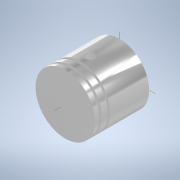
# Autodesk Inventor part: piston
Saved by Autodesk Inventor 2021.1 (Build 251245000, 245)
## iProperties
Created: 2020-08-31
Part Number: piston
Material: Aluminum 6061
Document SubType Name: Sheet Metal
Designer: Vamshi
Mass: 612.77 g
Surface Area: 445.688 cm^2
Volume: 226.952 cm^3
Density: 2.7 g/cm^3
Sheet Metal Rule: Default
Appearance: Aluminum - Flat
Author: Vamshi
Autodesk Inventor part; units mm, degrees
ref_plane "YZ Plane" through (0, 0, 0) normal (1, 0, 0) x (0, 1, 0)
ref_plane "XZ Plane" through (0, 0, 0) normal (0, 1, 0) x (-1, 0, 0)
ref_plane "XY Plane" through (0, 0, 0) normal (0, 0, 1) x (1, 0, 0)
sketch "Sketch1" plane through (0, 0, 0) normal (0, 0, 1) x (1, 0, 0)
  circle A0 centre (0, 0) radius 40.64
  dimension "d0" = 81.28
  constraints: 1 centre point, 1 coincident
  measures "d0" diameter of A0
extrude "Extrusion1" add sketch "Sketch1" along normal blind 81.28
sketch "Sketch2" plane through (0, 0, 0) normal (0, 1, 0) x (-1, 0, 0)
  line L0 (0, -16.256) -> (0, 97.536) construction
  line L1 (40.64, 81.28) -> (40.64, 0) construction
  line L2 (40.64, 0) -> (-40.64, 0) construction
  line L3 (-40.64, 0) -> (-40.64, 81.28) construction
  line L4 (-40.64, 81.28) -> (40.64, 81.28) construction
  line L5 (40.64, 81.28) -> (40.64, 0) construction
  line L6 (40.64, 0) -> (-40.64, 0) construction
  line L7 (-40.64, 0) -> (-40.64, 81.28) construction
  line L8 (-40.64, 81.28) -> (40.64, 81.28) construction
  line L9 (40.64, 81.28) -> (-40.64, 81.28) construction
  line L10 (40.64, 0) -> (-40.64, 0) construction
  line L11 (40.64, 0) -> (40.64, 81.28) projected
  line L12 (40.64, 68.58) -> (36.83, 68.58)
  line L13 (36.83, 68.58) -> (36.83, 64.77)
  line L14 (36.83, 64.77) -> (40.64, 64.77)
  line L15 (40.64, 64.77) -> (40.64, 68.58)
  line L16 (40.64, 57.15) -> (36.83, 57.15)
  line L17 (36.83, 57.15) -> (36.83, 53.34)
  line L18 (36.83, 53.34) -> (40.64, 53.34)
  line L19 (40.64, 53.34) -> (40.64, 57.15)
  line L20 (40.64, 0) -> (40.64, 81.28) projected
  line L21 (40.64, 81.28) -> (-40.64, 81.28) projected
  line L22 (0, 81.28) -> (40.64, 74.1141)
  line L23 (0, 0) -> (33.02, 0)
  line L24 (33.02, 0) -> (33.02, 25.4)
  line L25 (33.02, 25.4) -> (0, 25.4)
  line L26 (0, 25.4) -> (0, 0)
  line L27 (0, 25.4) -> (25.4, 25.4)
  line L28 (25.4, 25.4) -> (25.4, 60.96)
  line L29 (25.4, 60.96) -> (0, 60.96)
  line L30 (0, 60.96) -> (0, 25.4)
  dimension "d3" = 7.62
  dimension "d4" = 53.34
  dimension "d5" = 36.83
  dimension "d6" = 36.83
  dimension "d7" = 10
  dimension "d8" = 33.02
  dimension "d9" = 25.4
  dimension "d10" = 25.4
  dimension "d11" = 35.56
  dimension "d23" = 3.81
  dimension "d24" = 3.81
  constraints: 34 end point, 8 parallel, 4 horizontal, 4 perpendicular, 3 point on line, 1 midpoint, 2 other
  measures "d3" distance from line of L16.end L14
  measures "d4" distance from line of L1.end L18
  measures "d5" distance between parallel lines of L0 L13
  measures "d6" distance between parallel lines of L0 L17
  measures "d7" angle of L4 L22
  measures "d8" distance of L25.end L24.end
  measures "d9" distance of L24.end L23.end
  measures "d10" distance of L29.end L28.end
  measures "d11" distance of L28.end L27.end
  measures "d23" distance between parallel lines of L14 L12
  measures "d24" distance between parallel lines of L18 L16
revolve "Revolution1" cut sketch "Sketch2" angle 360 about axis through (0, 0, -10) along (0, 0, 1)
sketch "Sketch4" plane through (0, 0, 0) normal (0, 1, 0) x (-1, 0, 0)
  line L0 (0, 81.28) -> (40.64, 74.1141) projected
  line L1 (40.64, 74.1141) -> (40.64, 68.58) projected
  line L2 (40.64, 68.58) -> (36.83, 68.58) projected
  line L3 (36.83, 68.58) -> (36.83, 64.77) projected
  line L4 (36.83, 64.77) -> (40.64, 64.77) projected
  line L5 (40.64, 64.77) -> (40.64, 57.15) projected
  line L6 (40.64, 57.15) -> (36.83, 57.15) projected
  line L7 (36.83, 57.15) -> (36.83, 53.34) projected
  line L8 (36.83, 53.34) -> (40.64, 53.34) projected
  line L9 (40.64, 53.34) -> (40.64, 0) projected
  line L10 (40.64, 0) -> (33.02, 0) projected
  line L11 (33.02, 0) -> (33.02, 25.4) projected
  line L12 (33.02, 25.4) -> (25.4, 25.4) projected
  line L13 (25.4, 25.4) -> (25.4, 60.96) projected
  line L14 (25.4, 60.96) -> (-25.4, 60.96) projected
  line L15 (-25.4, 60.96) -> (-25.4, 25.4) projected
  line L16 (-25.4, 25.4) -> (-33.02, 25.4) projected
  line L17 (-33.02, 25.4) -> (-33.02, 0) projected
  line L18 (-33.02, 0) -> (-40.64, 0) projected
  line L19 (-40.64, 0) -> (-40.64, 53.34) projected
  line L20 (-40.64, 53.34) -> (-36.83, 53.34) projected
  line L21 (-36.83, 53.34) -> (-36.83, 57.15) projected
  line L22 (-36.83, 57.15) -> (-40.64, 57.15) projected
  line L23 (-40.64, 57.15) -> (-40.64, 64.77) projected
  line L24 (-40.64, 64.77) -> (-36.83, 64.77) projected
  line L25 (-36.83, 64.77) -> (-36.83, 68.58) projected
  line L26 (-36.83, 68.58) -> (-40.64, 68.58) projected
  line L27 (-40.64, 68.58) -> (-40.64, 74.1141) projected
  line L28 (-40.64, 74.1141) -> (0, 81.28) projected
  line L29 (-40.64, 74.1141) -> (40.64, 74.1141) projected
  line L30 (40.64, 74.1141) -> (0, 81.28) projected
  line L31 (-40.64, 74.1141) -> (0, 81.28) projected
  arc A0 (7.7717, 79.9096) -> (-7.7788, 79.9084) centre (0.0005, 29.7076) ccw
  line L32 (0, 81.28) -> (0, 80.5076)
  line L33 (0, -16.256) -> (0, 97.536) projected
  point P0 (0, 0)
  point P1 (-7.7788, 79.9084)
  dimension "d17" = 50.8
  constraints: 3 point on circle, 2 end point, 2 point on line, 1 centre point, 1 vertical
  measures "d17" radius of A0
revolve "Revolution2" cut sketch "Sketch4" angle 360 about axis through (0, 0, -10) along (0, 0, 1) contours L32 A0 L28
sketch "Sketch5" plane through (0, 0, 0) normal (0, 1, 0) x (-1, 0, 0)
  line L0 (-36.83, 53.34) -> (-36.83, 57.15) projected
  line L1 (-36.83, 57.15) -> (-40.64, 57.15) projected
  line L2 (-40.64, 57.15) -> (-40.64, 64.77) projected
  line L3 (-40.64, 64.77) -> (-36.83, 64.77) projected
  line L4 (-36.83, 64.77) -> (-36.83, 68.58) projected
  line L5 (-36.83, 68.58) -> (-40.64, 68.58) projected
  line L6 (-40.64, 68.58) -> (-40.64, 74.1141) projected
  line L7 (-40.64, 74.1141) -> (-7.7788, 79.9084) projected
  arc A0 (0, 80.5076) -> (-7.7788, 79.9084) centre (0.0005, 29.7076) ccw projected
  arc A1 (7.7788, 79.9084) -> (0, 80.5076) centre (-0.0005, 29.7076) ccw projected
  line L8 (7.7788, 79.9084) -> (40.64, 74.1141) projected
  line L9 (40.64, 74.1141) -> (40.64, 68.58) projected
  line L10 (40.64, 68.58) -> (36.83, 68.58) projected
  line L11 (36.83, 68.58) -> (36.83, 64.77) projected
  line L12 (36.83, 64.77) -> (40.64, 64.77) projected
  line L13 (40.64, 64.77) -> (40.64, 57.15) projected
  line L14 (40.64, 57.15) -> (36.83, 57.15) projected
  line L15 (36.83, 57.15) -> (36.83, 53.34) projected
  line L16 (36.83, 53.34) -> (40.64, 53.34) projected
  line L17 (40.64, 53.34) -> (40.64, 0) projected
  line L18 (40.64, 0) -> (33.02, 0) projected
  line L19 (33.02, 0) -> (33.02, 25.4) projected
  line L20 (33.02, 25.4) -> (25.4, 25.4) projected
  line L21 (25.4, 25.4) -> (25.4, 60.96) projected
  line L22 (25.4, 60.96) -> (-25.4, 60.96) projected
  line L23 (-25.4, 60.96) -> (-25.4, 25.4) projected
  line L24 (-25.4, 25.4) -> (-33.02, 25.4) projected
  line L25 (-33.02, 25.4) -> (-33.02, 0) projected
  line L26 (-33.02, 0) -> (-40.64, 0) projected
  line L27 (-40.64, 0) -> (-40.64, 53.34) projected
  line L28 (-40.64, 53.34) -> (-36.83, 53.34) projected
  line L29 (-7.7788, 79.9084) -> (7.7788, 79.9084) projected
  line L30 (-40.64, 74.1141) -> (40.64, 74.1141) projected
  line L31 (40.64, 68.58) -> (-40.64, 68.58) projected
  line L32 (-40.64, 74.1141) -> (40.64, 74.1141) projected
  line L33 (-40.64, 64.77) -> (40.64, 64.77) projected
  line L34 (-40.64, 53.34) -> (40.64, 53.34) projected
  line L35 (40.64, 0) -> (-40.64, 0) projected
  circle A2 centre (0, 40.64) radius 6.35
  point P0 (0, 0)
  dimension "d19" = 12.7
  dimension "d20" = 40.64
  constraints: 1 centre point
  measures "d19" diameter of A2
  measures "d20" distance of point (0, 0) A2.centre
extrude "Extrusion3" cut sketch "Sketch5" against normal through all both and the other way through all contours A2
equation "\"BendRadius\" = Thickness"
equation "\"BendReliefWidth\" = Thickness"
equation "\"BendReliefDepth\" = 0.5 * Thickness"
equation "\"CornerReliefSize\" = 4 * Thickness"
equation "\"MinimumRemnant\" = 2 * Thickness"
equation "\"TransitionRadius\" = BendRadius"
equation "\"JacobiRadiusSize\" = BendRadius"
equation "\"GapSize\" = Thickness"
equation "\"Thickness\" = 3.048"
body "Solid1"
